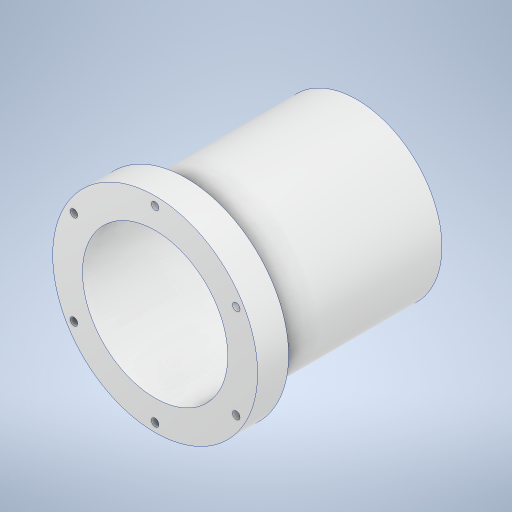
# Autodesk Inventor part: aluminium outer wall back
Saved by Autodesk Inventor 2023 (Build 270158000, 158)
## iProperties
Created: 2022-09-19
Part Number: aluminium outer wall back
Material: Aluminum 6061
Document SubType Name: Modeling
Designer: station
Density: 2.7 g/cm^3
Appearance: Aluminum - Flat
Author: station
Autodesk Inventor part; units mm, degrees
ref_plane "YZ Plane" through (0, 0, 0) normal (1, 0, 0) x (0, 1, 0)
ref_plane "XY Plane" through (0, 0, 0) normal (0, 0, 1) x (1, 0, 0)
sketch "Sketch1" plane through (0, 0, 0) normal (0, 0, 1) x (1, 0, 0)
  circle A0 centre (0, 0) radius 58.5
  circle A1 centre (0, 0) radius 68.5
  dimension "d0" = 117
  dimension "d1" = 137
  constraints: 2 centre point, 2 coincident
  measures "d0" diameter of A0
  measures "d1" diameter of A1
extrude "Extrusion1" add sketch "Sketch1" along normal blind 323.123
ref_plane "Work Plane1" through (0, 61.5, 0) normal (0, 1, 0) x (-1, 0, 0)
sketch "Sketch2" plane through (0, 61.5, 0) normal (0, 1, 0) x (-1, 0, 0)
  line L0 (68.5, 0) -> (-68.5, 0) projected
  line L1 (0, 0) -> (0, 4)
  line L2 (0, 4) -> (0, 8.666)
  circle A0 centre (0, 15.524) radius 6.858
  circle A1 centre (0, 15.524) radius 7.858
  dimension "d6" = 4
  dimension "d7" = 4.666
  dimension "d8" = 13.716
  dimension "d9" = 6.858
  dimension "d33" = 15.716
  constraints: 4 end point, 2 centre point, 1 coincident, 1 point on line, 1 vertical
  measures "d6" distance of L1.start L1.end
  measures "d7" distance of L1.end L2.end
  measures "d8" diameter of A0
  measures "d9" distance of A0.centre L2.end
  measures "d33" diameter of A1
sketch "Sketch4" plane through (0, 61.5, 0) normal (0, 1, 0) x (-1, 0, 0)
  point P0 (0, 0)
sketch "Sketch5" plane through (0, 61.5, 0) normal (0, 1, 0) x (-1, 0, 0)
  line L0 (0, 0) -> (0, 76) construction
  circle A0 centre (0, 76) radius 4
  dimension "d21" = 76
  dimension "d22" = 8
  constraints: 2 end point, 1 centre point, 1 coincident, 1 vertical
  measures "d21" distance of L0.start L0.end
  measures "d22" diameter of A0
extrude "Extrusion4" cut sketch "Sketch5" against normal through all
thread "Thread3" size "M8x1.25" class "6H" standard "ANSI Metric M Profile" full length
thread "Thread4" size "M8x1.25" class "6H" standard "ANSI Metric M Profile" full length
sketch "Sketch6" plane through (0, 0, 323.123) normal (0, 0, 1) x (1, 0, 0)
  circle A0 centre (0, 0) radius 75
  circle A1 centre (0, 0) radius 61.5
  dimension "d29" = 150
  dimension "d30" = 123
  constraints: 2 centre point, 2 coincident
  measures "d29" diameter of A0
  measures "d30" diameter of A1
extrude "Extrusion5" add sketch "Sketch6" against normal blind 2
ref_plane "Work Plane2" through (0, 0, 162.5) normal (0, 0, -1) x (-1, 0, 0)
sketch "Sketch7" plane through (0, 0, 162.5) normal (0, 0, -1) x (-1, 0, 0)
  circle A0 centre (0, 0) radius 58.5 projected
  circle A1 centre (0, 0) radius 65.45
  circle A2 centre (0, 0) radius 75 construction
  circle A3 centre (0, 0) radius 75.5
  circle A4 centre (0, 0) radius 82.5
  circle A5 centre (0, 0) radius 79.5 construction
  circle A6 centre (0, 0) radius 75.5
  circle A7 centre (0, 75.5) radius 3
  circle A8 centre (-65.3849, 37.75) radius 3
  circle A9 centre (-65.3849, -37.75) radius 3
  circle A10 centre (0, -75.5) radius 3
  circle A11 centre (65.3849, -37.75) radius 3
  circle A12 centre (65.3849, 37.75) radius 3
  point P0 (66.3756, 34.9183)
  point P1 (63.4279, 40.0238)
  point P2 (2.9477, 74.9421)
  point P3 (-2.9477, 74.9421)
  point P4 (-63.4279, 40.0238)
  point P5 (-66.3756, 34.9183)
  point P6 (-66.3756, -34.9183)
  point P7 (-63.4279, -40.0238)
  point P8 (-2.9477, -74.9421)
  point P9 (2.9477, -74.9421)
  point P10 (63.4279, -40.0238)
  point P11 (66.3756, -34.9183)
  point P12 (63.8336, 40.3178)
  point P13 (66.833, 35.1226)
  point P14 (66.833, -35.1226)
  point P15 (63.8336, -40.3178)
  point P16 (2.9994, -75.4404)
  point P17 (-2.9994, -75.4404)
  point P18 (-63.8336, -40.3178)
  point P19 (-66.833, -35.1226)
  point P20 (-66.833, 35.1226)
  point P21 (-63.8336, 40.3178)
  point P22 (-2.9994, 75.4404)
  point P23 (2.9994, 75.4404)
  dimension "d80" = 151
  dimension "d93" = 165
  dimension "d94" = 159
  dimension "d95" = 151
  dimension "d96" = 6
  dimension "d99" = 360
  constraints: 10 centre point, 6 coincident, 16 other
  measures "d93" diameter of A4
  measures "d94" diameter of A5
  measures "d95" diameter of A6
  measures "d96" diameter of A7
split "Split3" plane through (0, 0, 162.5) removes the side toward (0, 0, 1)
hole "Hole2" at (0, 61.5, 15.524) direction (0, -1, 0) diameter 13.716 end up to face face through (0, 0, 0) facing (0, 0, 1) round with radius 68.5 far side no
thread "Thread5" size "M14x2" class "6H" standard "ANSI Metric M Profile" full length
hole "Hole4" at (0, 75.5, 162.5) direction (0, 0, -1) diameter 6 end through all
extrude "Extrusion12" add sketch "Sketch7" along normal blind 25 contours A1 | A3 A11 A10 A9 A8 A7 A12 | A4
body "Solid1"
